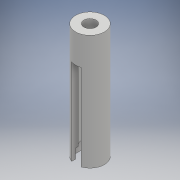
# Autodesk Inventor part: Rotation
Saved by Autodesk Inventor 2018 (Build 220112000, 112)
## iProperties
Created: 2019-07-18
Part Number: Rotation
Material: Generic
Document SubType Name: Modeling
Designer: aal_9
Density: 1 g/cm^3
Appearance: Default
Author: aal_9
Autodesk Inventor part; units mm, degrees
ref_plane "YZ Plane" through (0, 0, 0) normal (1, 0, 0) x (0, 1, 0)
ref_plane "XY Plane" through (0, 0, 0) normal (0, 0, 1) x (1, 0, 0)
sketch "Sketch1" plane through (0, 0, 0) normal (0, 0, 1) x (1, 0, 0)
  circle A0 centre (0, 0) radius 4.45
  circle A1 centre (0, 0) radius 7.5
  dimension "d0" = 8.9
  dimension "d1" = 15
  constraints: 2 centre point, 2 coincident
  measures "d0" diameter of A0
  measures "d1" diameter of A1
extrude "Extrusion1" add sketch "Sketch1" along normal blind 60
ref_plane "Work Plane1" through (0, 7.5, 0) normal (0, 1, 0) x (-1, 0, 0)
sketch "Sketch2" plane through (0, 7.5, 0) normal (0, 1, 0) x (-1, 0, 0)
  line L0 (2.5, 45) -> (-2.5, 45)
  line L1 (-2.5, 45) -> (-2.5, 0)
  line L2 (-2.5, 0) -> (2.5, 0)
  line L3 (2.5, 0) -> (2.5, 45)
  line L4 (7.5, 60) -> (-7.5, 60) projected
  line L5 (-7.5, 0) -> (7.5, 0) projected
  point P0 (0, 0)
  dimension "d4" = 45
  dimension "d6" = 5
  dimension "d7" = 2.5
  dimension "d22" = 0
  constraints: 8 end point, 2 parallel, 1 horizontal, 1 perpendicular
  measures "d4" distance of L0.end L1.end
  measures "d6" distance of L1.end L2.end
  measures "d7" distance from line of point (0, 0) L3
  measures "d22" distance between parallel lines of L5 L2
extrude "Extrusion2" cut sketch "Sketch2" against normal through all
sketch "Sketch3" plane through (0, 0, 60) normal (0, 0, 1) x (1, 0, 0)
  circle A0 centre (0, 0) radius 3.2
  circle A1 centre (0, 0) radius 4.45
  dimension "d10" = 6.4
  constraints: 2 centre point, 2 coincident
  measures "d10" diameter of A0
extrude "Extrusion3" add sketch "Sketch3" against normal blind 10
sketch "Sketch4" plane through (0, 0, 0) normal (0, 0, -1) x (-1, 0, 0)
  circle A0 centre (0, 0) radius 4.45
  constraints: 1 centre point, 1 coincident
extrude "Extrusion4" add sketch "Sketch4" against normal blind 5
sketch "Sketch5" plane through (0, 0, 0) normal (0, 0, -1) x (0, -1, 0)
  line L0 (-5, -5) -> (5, -5)
  line L1 (5, -5) -> (5, 5)
  line L2 (5, 5) -> (-5, 5)
  line L3 (-5, 5) -> (-5, -5)
  point P0 (0, 0)
  dimension "d16" = 10
  dimension "d17" = 5
  dimension "d18" = 10
  dimension "d19" = 5
  constraints: 8 end point, 2 parallel, 1 horizontal, 1 perpendicular
  measures "d16" distance of L0.end L1.end
  measures "d17" distance from line of point (0, 0) L0
  measures "d18" distance between parallel lines of L1 L3
  measures "d19" distance from line of point (0, 0) L3
extrude "Extrusion5" cut sketch "Sketch5" against normal blind 5
equation "\"d17\" = 0.5 * d16"
equation "\"d19\" = 0.5 * d18"
body "Solid1"
